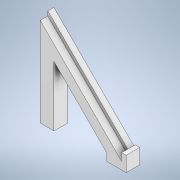
# Autodesk Inventor part: BaseBeamSplitter-D
Saved by Autodesk Inventor 2022.2 (Build 262287010, 287A)
## iProperties
Created: 2022-04-08
Part Number: BaseBeamSplitter-D
Material: Plástico ABS
Document SubType Name: Modeling
Designer: mabel
Density: 1.06 g/cm^3
Appearance: Suave - Blanco
Author: mabel
Autodesk Inventor part; units mm, degrees
ref_plane "YZ Plane" through (0, 0, 0) normal (1, 0, 0) x (0, 1, 0)
ref_plane "XZ Plane" through (0, 0, 0) normal (0, 1, 0) x (-1, 0, 0)
ref_plane "XY Plane" through (0, 0, 0) normal (0, 0, 1) x (1, 0, 0)
sketch "Boceto1" plane through (0, 0, 0) normal (0, 0, 1) x (1, 0, 0)
  line L0 (-9.0701, 0) -> (44.9299, 0)
  line L1 (44.9299, 0) -> (-9.0701, 54)
  line L2 (-9.0701, 0) -> (-9.0701, 54)
  point P0 (0, 0)
  dimension "d0" = 54
  dimension "d2" = 45
  constraints: 6 end point, 1 horizontal, 1 vertical
  measures "d0" distance of L0.start L0.end
  measures "d2" angle of L1 L0
extrude "Extrusión1" add sketch "Boceto1" along normal blind 5
sketch "Boceto2" plane through (0, 0, 5) normal (0, 0, 1) x (1, 0, 0)
  line L0 (44.9299, 0) -> (-9.0701, 54) projected
  line L1 (44.9299, 5) -> (47.9299, 5)
  line L2 (47.9299, 5) -> (47.9299, 0)
  line L3 (47.9299, 0) -> (44.9299, 0)
  line L4 (44.9299, 0) -> (44.9299, 5)
  point P0 (0, 0)
  dimension "d9" = 3
  dimension "d10" = 5
  constraints: 8 end point, 2 parallel, 1 horizontal, 1 perpendicular
  measures "d9" distance of L2.end L3.end
  measures "d10" distance of L1.end L2.end
extrude "Extrusión2" add sketch "Boceto2" against normal blind 9
sketch "Boceto4" plane through (0, 0, 0) normal (0, 0, -1) x (-1, 0, 0)
  line L0 (-48.0778, 0) -> (35.3608, 0) construction
  line L1 (-47.9299, 5) -> (-47.9299, 0) projected
  line L2 (-47.9299, 0) -> (9.0701, 57)
  line L3 (-47.9299, 0) -> (40.6563, 0) construction
  line L4 (9.0701, 0) -> (9.0701, 57)
  line L5 (9.0701, 0) -> (-47.9299, 0)
  point P0 (0, 0)
  dimension "d24" = 45
  constraints: 10 end point, 2 horizontal, 1 collinear, 1 vertical
  measures "d24" angle of L3 L2
extrude "Extrusión3" add sketch "Boceto4" along normal blind 4
sketch "Boceto5" plane through (0, 0, -4) normal (0, 0, -1) x (-1, 0, 0)
  line L0 (0, 0) -> (0, 35)
  line L1 (0, 35) -> (-35, 0)
  line L2 (0, 35) -> (67.1316, 35) construction
  line L3 (0, 0) -> (-35, 0)
  line L4 (9.0701, 0) -> (-44.9299, 0) projected
  dimension "d19" = 35
  dimension "d20" = 135
  constraints: 8 end point, 1 horizontal, 1 point on line, 1 vertical
  measures "d19" distance of L0.start L0.end
  measures "d20" angle of L1 L2
extrude "Extrusión4" cut sketch "Boceto5" against normal blind 15
sketch "Boceto6" plane through (-9.0701, 0, -4) normal (0, -1, 0) x (1, 0, 0)
  line L0 (9.0701, 0) -> (9.0701, 9) projected
  line L1 (9.0701, 9) -> (0, 9)
  line L2 (0, 9) -> (0, 0)
  line L3 (0, 0) -> (9.0701, 0)
  line L4 (9.0701, 0) -> (9.0701, 9)
  point P0 (9.0701, 4)
  constraints: 8 end point, 2 parallel, 1 horizontal, 1 perpendicular
extrude "Extrusión5" add sketch "Boceto6" along normal blind 5
sketch "Boceto7" plane through (44.9299, 0, 5) normal (0, -1, 0) x (1, 0, 0)
  line L0 (-9.9299, -9) -> (-44.9299, -9) projected
  line L1 (3, 0) -> (0, 0) projected
  line L2 (-9.9299, -9) -> (3, -9)
  line L3 (3, -9) -> (3, 0)
  line L4 (3, 0) -> (-9.9299, 0)
  line L5 (-9.9299, 0) -> (-9.9299, -9)
  point P0 (-44.9299, -5)
  constraints: 8 end point, 2 parallel, 1 horizontal, 1 perpendicular
extrude "Extrusión6" add sketch "Boceto7" along normal blind 5
ref_plane "Plano de trabajo1" through (0, 0, 16) normal (0, 0, 1) x (1, 0, 0)
